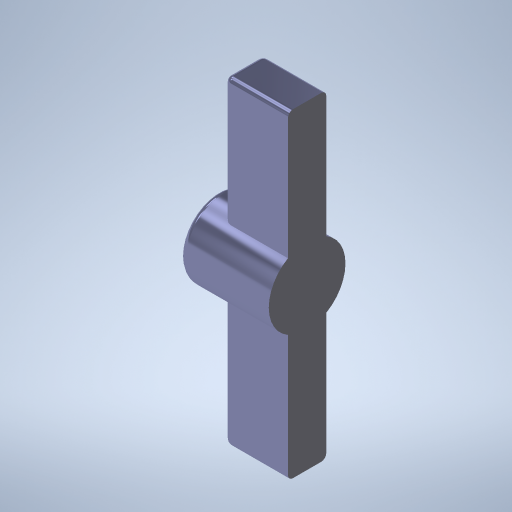
# Autodesk Inventor part: torque
Saved by Autodesk Inventor 2023 (Build 270158000, 158)
## iProperties
Created: 2022-11-03
Part Number: torque
Material: Generic
Document SubType Name: Modeling
Designer: Xiaba
Density: 1 g/cm^3
Appearance: Default
Author: Xiaba
Autodesk Inventor part; units mm, degrees
ref_plane "YZ Plane" through (0, 0, 0) normal (1, 0, 0) x (0, 1, 0)
ref_plane "XZ Plane" through (0, 0, 0) normal (0, 1, 0) x (-1, 0, 0)
ref_plane "XY Plane" through (0, 0, 0) normal (0, 0, 1) x (1, 0, 0)
sketch "Sketch1" plane through (0, 0, 0) normal (1, 0, 0) x (0, 1, 0)
  line L0 (13.9123, 0.5821) -> (-10.2877, 0.5821)
  line L1 (-10.6877, 0.1821) -> (-10.6877, -2.0179)
  line L2 (-10.2877, -2.4179) -> (13.9123, -2.4179)
  line L3 (14.3123, -2.0179) -> (14.3123, 0.1821)
  arc A0 (13.9123, -2.4179) -> (14.3123, -2.0179) centre (13.9123, -2.0179) ccw
  arc A1 (14.3123, 0.1821) -> (13.9123, 0.5821) centre (13.9123, 0.1821) ccw
  arc A2 (-10.6877, -2.0179) -> (-10.2877, -2.4179) centre (-10.2877, -2.0179) ccw
  arc A3 (-10.2877, 0.5821) -> (-10.6877, 0.1821) centre (-10.2877, 0.1821) ccw
  line L4 (14.3123, -4.8123) -> (1.8123, -4.8123) construction
  line L5 (14.3123, 0.1821) -> (14.3123, -23.1695) construction
  circle A4 centre (1.8123, -0.9179) radius 3
  circle A5 centre (1.8123, -0.9179) radius 1.5
  point P0 (0, 0)
  point P1 (-10.6877, -2.4179)
  point P2 (-10.6877, 0.5821)
  point P3 (14.3123, -2.4179)
  point P4 (4.4103, 0.5821)
  point P5 (-0.7858, 0.5821)
  point P6 (-0.7858, -2.4179)
  point P7 (4.4103, -2.4179)
  dimension "d1" = 3
  dimension "d2" = 25
  dimension "d3" = 0.4
  dimension "d4" = 12.5
  dimension "d5" = 6
  constraints: 12 end point, 9 tangent, 8 point on circle, 7 point on line, 6 centre point, 3 equal radius, 2 horizontal, 2 parallel, 1 coincident, 1 perpendicular, 1 vertical
  measures "d1" distance of point (-10.688, 0.582) point (-10.688, -2.418)
  measures "d2" distance of point (-10.688, -2.418) point (14.312, -2.418)
  measures "d3" radius of A0
  measures "d4" distance of L4.start L4.end
  measures "d5" diameter of A4
extrude "Extrusion1" add sketch "Sketch1" along normal blind 2
extrude "Extrusion2" add sketch "Sketch1" against normal blind 2 contours A4 L2 A5 L0 | L0 A4 | A5 L2 A4 L0 | A5 | L2 A4
extrude "Extrusion3" add sketch "Sketch1" against normal blind 3 contours A5
fillet "Fillet1" radius 0.5 1 edges at (-3, 0.3123, -0.9179)
fillet "Fillet2" radius 0.5 1 edges at (-2, -1.1877, -0.9179)
fillet "Fillet3" radius 0.5 10 edges at (0, 14.1951, 0.465) (0, 14.3123, -0.9179) (0, 14.1951, -2.3007) (0, 9.1613, -2.4179) (0, 9.1613, 0.5821) (0, -10.5706, 0.465) (0, -10.6877, -0.9179) (0, -10.5706, -2.3007) (0, -5.5368, -2.4179) (0, -5.5368, 0.5821)
sketch "Sketch2" plane through (2, 0, 0) normal (1, 0, 0) x (0, 0, -1)
  line L0 (-0.5821, 13.9123) -> (-0.5821, 4.4103) projected
  arc A0 (-0.5821, 4.4103) -> (-0.5821, -0.7858) centre (0.9179, 1.8123) ccw projected
  line L1 (-0.5821, -0.7858) -> (-0.5821, -10.2877) projected
  arc A1 (-0.5821, -10.2877) -> (-0.1821, -10.6877) centre (-0.1821, -10.2877) ccw projected
  line L2 (-0.1821, -10.6877) -> (2.0179, -10.6877) projected
  arc A2 (2.0179, -10.6877) -> (2.4179, -10.2877) centre (2.0179, -10.2877) ccw projected
  line L3 (2.4179, -10.2877) -> (2.4179, -0.7858) projected
  arc A3 (2.4179, -0.7858) -> (2.4179, 4.4103) centre (0.9179, 1.8123) ccw projected
  line L4 (2.4179, 4.4103) -> (2.4179, 13.9123) projected
  arc A4 (2.4179, 13.9123) -> (2.0179, 14.3123) centre (2.0179, 13.9123) ccw projected
  line L5 (2.0179, 14.3123) -> (-0.1821, 14.3123) projected
  arc A5 (-0.1821, 14.3123) -> (-0.5821, 13.9123) centre (-0.1821, 13.9123) ccw projected
  point P0 (0, 0)
extrude "Extrusion4" add sketch "Sketch2" along normal blind 3
body "Solid1"
